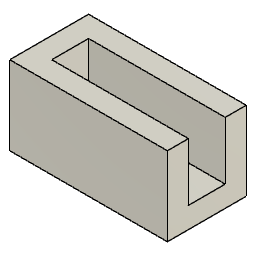
sorted_smarties_cover_connector_base (Autodesk Fusion 360 design; units mm, degrees)
Autodesk Fusion 360 part; units mm, degrees
sketch "Sorted Smarties Cover Connector Base" plane through (0, 0, 0) normal (0, 0, 1) x (1, 0, 0)
  line L0 (0, 0) -> (30, 0)
  line L1 (30, 0) -> (30, 15)
  line L2 (30, 15) -> (0, 15)
  line L3 (0, 15) -> (0, 0)
  dimension "d5" = 15
  dimension "d6" = 30
  constraint horizontal L0
  constraint vertical L1
  constraint horizontal L2
  constraint vertical L3
  constraint coincident L0.start L3.end
  measures "d5" distance of L0.start L2.end
  measures "d6" distance of L0.start L0.end
extrude "Extrude1" add sketch "Sorted Smarties Cover Connector Base" along normal blind 15
sketch "Connecting Section" plane through (0, 0, 15) normal (0, 0, 1) x (-1, 0, 0)
  line L0 (0, -15) -> (0, 0)
  line L1 (0, 0) -> (-30, 0)
  line L2 (-30, 0) -> (-30, -15)
  line L3 (-30, -15) -> (0, -15)
  line L4 (-30, -11) -> (-4, -11)
  line L5 (-4, -11) -> (-4, -4)
  line L6 (-4, -4) -> (-30, -4)
  line L7 (-30, -4) -> (-30, -11)
  dimension "d7" = 7
  dimension "d8" = 4
  dimension "d9" = 4
  dimension "d10" = 4
  constraint horizontal L4
  constraint vertical L5
  constraint horizontal L6
  constraint vertical L7
  constraint coincident L2 L4.start
  measures "d7" distance of L4 L6
  measures "d8" distance of L1 L6
  measures "d9" distance of L3 L4
  measures "d10" distance of L0 L5
extrude "Extrude2" cut sketch "Connecting Section" against normal blind 11 contours L2 L4 L5 L6 L7
equation "d8 = ( ( 15 - 7 ) / 2 ) * 1 mm"
named bodies: "Sorted Smarties Cover Connector Base"
